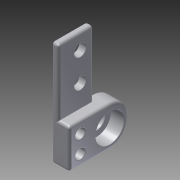
# Autodesk Inventor part: 13mmBearingBracketRight
Saved by Autodesk Inventor 2015 (Build 190159000, 159)
## iProperties
Created: 2013-07-06
Part Number: 13mmBearingBracketRight
Material: Generic
Document SubType Name: Modeling
Designer: mhgreen
Density: 1 g/cm^3
Appearance: Default
Author: mhgreen
Autodesk Inventor part; units mm, degrees
ref_plane "YZ Plane" through (0, 0, 0) normal (1, 0, 0) x (0, 1, 0)
ref_plane "XZ Plane" through (0, 0, 0) normal (0, 1, 0) x (-1, 0, 0)
ref_plane "XY Plane" through (0, 0, 0) normal (0, 0, 1) x (1, 0, 0)
sketch "Sketch1" plane through (0, 0, 0) normal (1, 0, 0) x (0, 1, 0)
  line L0 (27, 0) -> (27, -18)
  line L1 (0, 0) -> (0, -18)
  line L2 (27, -18) -> (0, -18)
  line L3 (0, 0) -> (27, 0)
  dimension "d0" = 18
  dimension "d2" = 27
  constraints: 8 end point, 1 parallel
  measures "d0" distance of L0.start L0.end
  measures "d2" distance of L1.start L0.start
sketch "Sketch2" plane through (0, 0, 0) normal (1, 0, 0) x (0, 1, 0)
  line L0 (16, 30) -> (0, 30)
  line L1 (0, 30) -> (0, 0)
  line L2 (16, 0) -> (16, 30)
  line L3 (0, 0) -> (16, 0)
  dimension "d3" = 16
  dimension "d4" = 30
  constraints: 8 end point, 2 parallel, 1 horizontal, 1 perpendicular, 1 vertical
  measures "d3" distance of L0.end L0.start
  measures "d4" distance of L0.start L2.start
extrude "Extrusion1" add sketch "Sketch2" along normal blind 3.25
extrude "Extrusion2" add sketch "Sketch1" along normal blind 8.25
sketch "Sketch4" plane through (3.25, 0, 0) normal (1, 0, 0) x (0, 0, -1)
  line L0 (-30, 16) -> (-30, 0) projected
  line L1 (-30, 0) -> (0, 0) projected
  line L2 (0, 0) -> (0, 16) projected
  point P0 (-23, 10)
  point P1 (-10, 10)
  dimension "d12" = 7
  dimension "d13" = 10
  dimension "d14" = 10
  dimension "d15" = 10
  measures "d12" distance from line of L0 point (-23, 10)
  measures "d13" distance from line of L2 point (-10, 10)
  measures "d14" distance from line of L1 point (-23, 10)
  measures "d15" distance from line of L1 point (-10, 10)
hole "Hole1" at (3.25, 10, 23) at (3.25, 10, 10) direction (-1, 0, 0) diameter 5.3 end through all
sketch "Sketch5" plane through (8.25, 0, 0) normal (1, 0, 0) x (0, 0, -1)
  line L0 (18, 27) -> (0, 27) projected
  line L1 (18, 0) -> (18, 27) projected
  point P0 (9.5, 18.5)
  dimension "d24" = 8.5
  dimension "d45" = 8.5
  measures "d24" distance from line of L0 point (9.5, 18.5)
  measures "d45" distance from line of L1 point (9.5, 18.5)
hole "Hole2" at (8.25, 18.5, -9.5) direction (-1, 0, 0) diameter 13.06 depth 6.1
sketch "Sketch6" plane through (0, 0, 0) normal (-1, 0, 0) x (0, 0, 1)
  line L0 (-18, 27) -> (0, 27) projected
  line L1 (-18, 0) -> (-18, 27) projected
  point P0 (0, 0)
  point P1 (-9.5, 18.5)
  dimension "d33" = 8.5
  dimension "d34" = 8.5
  measures "d33" distance from line of L0 point (-9.5, 18.5)
  measures "d34" distance from line of L1 point (-9.5, 18.5)
hole "Hole3" at (0, 18.5, -9.5) direction (1, 0, 0) diameter 8 end through all
fillet "Fillet1" radius 8.5 2 edges at (4.125, 27, 0) (4.125, 27, -18)
sketch "Sketch7" plane through (8.25, 0, 0) normal (1, 0, 0) x (0, 0, -1)
  line L0 (0, 18.5) -> (0, 0) projected
  line L1 (0, 0) -> (18, 0) projected
  line L2 (18, 0) -> (18, 18.5) projected
  point P0 (13, 5)
  point P1 (5, 5)
  point P2 (13, 5)
  point P3 (5, 5)
  dimension "d46" = 5
  dimension "d47" = 5
  dimension "d48" = 5
  dimension "d49" = 5
  constraints: 2 coincident
  measures "d46" distance from line of L2 point (13, 5)
  measures "d47" distance from line of L0 point (5, 5)
  measures "d48" distance from line of L1 point (5, 5)
  measures "d49" distance from line of L1 point (13, 5)
hole "Hole4" at (8.25, 5, -13) at (8.25, 5, -5) direction (-1, 0, 0) diameter 4.4 end through all
fillet "Fillet3" radius 0.25 11 edges at (3.25, 10, 25.65) (3.25, 10, 12.65) (8.25, 18.5, -2.97) (2.15, 18.5, -13.5) (0, 10, 25.65) (0, 10, 12.65) (0, 18.5, -13.5) (8.25, 5, -2.8) (8.25, 5, -10.8) (0, 5, -10.8) (0, 5, -2.8)
fillet "Fillet4" radius 1.2 20 edges at (8.25, 24.5104, -15.5104) (8.25, 27, -9) (8.25, 24.5104, -2.4896) (8.25, 9.25, 0) (8.25, 0, -9) (8.25, 9.25, -18) (0, 24.5104, -15.5104) (0, 9.25, -18) (0, 0, 6) (0, 8, 30) (0, 16, 15) (0, 24.5104, -2.4896) (0, 27, -9) (4.125, 0, -18) (5.75, 0, 0) (3.25, 0, 15) (1.625, 0, 30) (3.25, 16, 15) (3.25, 8, 30) (1.625, 16, 30)
body "Solid1"
